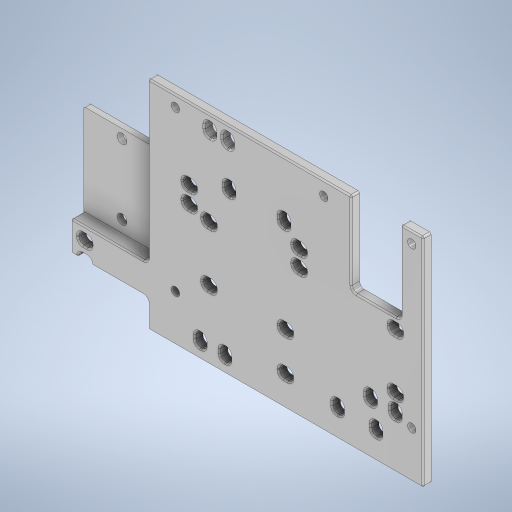
# Autodesk Inventor part: Cable_Fastener_10Gbit
Saved by Autodesk Inventor 2024 (Build 280153000, 153)
## iProperties
Created: 2020-06-16
Part Number: Cable_Fastener_10Gbit
Material: Generic
Document SubType Name: Modeling
Designer: Viktor Lindström
Density: 1 g/cm^3
Appearance: Default
Author: Viktor Lindström
Autodesk Inventor part; units mm, degrees
(part 1 of 2)
ref_plane "YZ Plane" through (0, 0, 0) normal (1, 0, 0) x (0, 1, 0)
ref_plane "XZ Plane" through (0, 0, 0) normal (0, 1, 0) x (-1, 0, 0)
ref_plane "XY Plane" through (0, 0, 0) normal (0, 0, 1) x (1, 0, 0)
sketch "Sketch1" plane through (0, 0, 0) normal (0, 0, 1) x (1, 0, 0)
  line L0 (-50, -39.5) -> (50, -39.5)
  line L1 (50, -39.5) -> (50, 39.5)
  line L2 (50, 39.5) -> (-50, 39.5)
  line L3 (-50, 39.5) -> (-50, -39.5)
  line L4 (-50, -39.5) -> (50, 39.5) construction
  line L5 (50, -39.5) -> (-50, 39.5) construction
  point P0 (0, 0)
  dimension "d0" = 100
  dimension "d1" = 79
  constraints: 12 end point, 2 midpoint, 2 parallel, 1 horizontal, 1 perpendicular
  measures "d0" distance of L1.end L2.end
  measures "d1" distance of L0.end L1.end
extrude "Extrusion1" add sketch "Sketch1" along normal blind 3
sketch "Sketch2" plane through (0, 0, 3) normal (0, 0, 1) x (1, 0, 0)
  circle A0 centre (-40, 35.5) radius 1.5
  circle A1 centre (46, 35.5) radius 1.5
  line L0 (50, 39.5) -> (-50, 39.5) projected
  line L1 (50, -39.5) -> (50, 39.5) projected
  line L2 (-73.7236, 6.5) -> (70.0965, 6.5) construction
  circle A2 centre (-40, -22.5) radius 1.5
  circle A3 centre (46, -22.5) radius 1.5
  point P0 (0, 0)
  dimension "d4" = 3
  dimension "d5" = 3
  dimension "d6" = 86
  dimension "d7" = 4
  dimension "d8" = 4
  dimension "d9" = 4
  dimension "d10" = 33
  constraints: 4 centre point, 2 end point, 2 symmetric about line, 1 horizontal, 2 other
  measures "d4" diameter of A0
  measures "d5" diameter of A1
  measures "d6" distance of A1.centre A0.centre
  measures "d7" distance from line of L0 A1.centre
  measures "d8" distance from line of L0 A0.centre
  measures "d9" distance from line of L1 A1.centre
  measures "d10" distance between parallel lines of L0 L2
extrude "Extrusion2" cut sketch "Sketch2" against normal through all
fillet "Fillet1" radius 0.6 4 edges at (50, 39.5, 1.5) (-50, 39.5, 1.5) (-50, -39.5, 1.5) (50, -39.5, 1.5)
sketch "Sketch3" plane through (0, 0, 3) normal (0, 0, 1) x (1, 0, 0)
  line L0 (31, -32) -> (35, -32)
  line L1 (35, -32) -> (35, -27)
  line L2 (35, -27) -> (31, -27)
  line L3 (31, -27) -> (31, -32)
  line L4 (31, -32) -> (35, -27) construction
  line L5 (35, -32) -> (31, -27) construction
  line L6 (21, -27) -> (17, -27)
  line L7 (17, -27) -> (17, -32)
  line L8 (17, -32) -> (21, -32)
  line L9 (21, -32) -> (21, -27)
  line L10 (21, -27) -> (17, -32) construction
  line L11 (17, -27) -> (21, -32) construction
  line L12 (-2.5, -30.5) -> (2.5, -30.5)
  line L13 (2.5, -30.5) -> (2.5, -26.5)
  line L14 (2.5, -26.5) -> (-2.5, -26.5)
  line L15 (-2.5, -26.5) -> (-2.5, -30.5)
  line L16 (-2.5, -30.5) -> (2.5, -26.5) construction
  line L17 (2.5, -30.5) -> (-2.5, -26.5) construction
  line L18 (-2.5, -12.5) -> (2.5, -12.5)
  line L19 (2.5, -12.5) -> (2.5, -16.5)
  line L20 (2.5, -16.5) -> (-2.5, -16.5)
  line L21 (-2.5, -16.5) -> (-2.5, -12.5)
  line L22 (-2.5, -12.5) -> (2.5, -16.5) construction
  line L23 (2.5, -12.5) -> (-2.5, -16.5) construction
  line L24 (-18.5, 17) -> (-22.5, 17)
  line L25 (-22.5, 17) -> (-22.5, 22)
  line L26 (-22.5, 22) -> (-18.5, 22)
  line L27 (-18.5, 22) -> (-18.5, 17)
  line L28 (-18.5, 17) -> (-22.5, 22) construction
  line L29 (-22.5, 17) -> (-18.5, 22) construction
  line L30 (1.5, 17) -> (-2.5, 17)
  line L31 (-2.5, 17) -> (-2.5, 22)
  line L32 (-2.5, 22) -> (1.5, 22)
  line L33 (1.5, 22) -> (1.5, 17)
  line L34 (1.5, 17) -> (-2.5, 22) construction
  line L35 (-2.5, 17) -> (1.5, 22) construction
  line L36 (37.5, 3.5) -> (42.5, 3.5)
  line L37 (42.5, 3.5) -> (42.5, 7.5)
  line L38 (42.5, 7.5) -> (37.5, 7.5)
  line L39 (37.5, 7.5) -> (37.5, 3.5)
  line L40 (37.5, 3.5) -> (42.5, 7.5) construction
  line L41 (42.5, 3.5) -> (37.5, 7.5) construction
  line L42 (-30.3047, -16.5) -> (-25.3047, -16.5)
  line L43 (-25.3047, -16.5) -> (-25.3047, -12.5)
  line L44 (-25.3047, -12.5) -> (-30.3047, -12.5)
  line L45 (-30.3047, -12.5) -> (-30.3047, -16.5)
  line L46 (-30.3047, -16.5) -> (-25.3047, -12.5) construction
  line L47 (-25.3047, -16.5) -> (-30.3047, -12.5) construction
  line L48 (-25.3047, 3.5) -> (-30.3047, 3.5)
  line L49 (-30.3047, 3.5) -> (-30.3047, 7.5)
  line L50 (-30.3047, 7.5) -> (-25.3047, 7.5)
  line L51 (-25.3047, 7.5) -> (-25.3047, 3.5)
  line L52 (-25.3047, 3.5) -> (-30.3047, 7.5) construction
  line L53 (-30.3047, 3.5) -> (-25.3047, 7.5) construction
  line L54 (50, -38.9) -> (50, 38.9) projected
  line L55 (-49.4, -39.5) -> (49.4, -39.5) projected
  line L56 (49.4, 39.5) -> (-49.4, 39.5) projected
  line L57 (42.5, -16.5) -> (37.5, -16.5)
  line L58 (37.5, -16.5) -> (37.5, -12.5)
  line L59 (37.5, -12.5) -> (42.5, -12.5)
  line L60 (42.5, -12.5) -> (42.5, -16.5)
  line L61 (42.5, -16.5) -> (37.5, -12.5) construction
  line L62 (37.5, -16.5) -> (42.5, -12.5) construction
  line L63 (-50, 38.9) -> (-50, -38.9) projected
  point P0 (0, 0)
  point P1 (33, -29.5)
  point P2 (19, -29.5)
  point P3 (0, -28.5)
  point P4 (0, -14.5)
  point P5 (-20.5, 19.5)
  point P6 (-0.5, 19.5)
  point P7 (40, 5.5)
  point P8 (-27.8047, -14.5)
  point P9 (-27.8047, 5.5)
  point P10 (40, -14.5)
  dimension "d14" = 4
  dimension "d15" = 4
  dimension "d16" = 4
  dimension "d17" = 4
  dimension "d18" = 4
  dimension "d19" = 4
  dimension "d20" = 4
  dimension "d21" = 4
  dimension "d23" = 4
  dimension "d24" = 5
  dimension "d25" = 5
  dimension "d26" = 5
  dimension "d27" = 5
  dimension "d29" = 5
  dimension "d30" = 5
  dimension "d31" = 5
  dimension "d32" = 5
  dimension "d33" = 5
  dimension "d34" = 0
  dimension "d35" = 20
  dimension "d36" = 20
  dimension "d37" = 14
  dimension "d38" = 14
  dimension "d40" = 17
  dimension "d41" = 10
  dimension "d42" = 25
  dimension "d43" = 50
  dimension "d44" = 34
  dimension "d45" = 4
  dimension "d46" = 5
  dimension "d47" = 20
  dimension "d48" = 0
  dimension "d49" = 0
  dimension "d50" = 10
  dimension "d125" = 20
  dimension "d126" = 29.5
  constraints: 120 end point, 20 midpoint, 20 parallel, 10 horizontal, 10 perpendicular, 3 point on line
  measures "d14" distance of L14.end L12.start
  measures "d15" distance of L18.end L19.end
  measures "d16" distance of L44.end L42.start
  measures "d17" distance of L48.end L49.end
  measures "d18" distance of L24.start L24.end
  measures "d19" distance of L30.start L30.end
  measures "d20" distance of L6.start L6.end
  measures "d21" distance of L1.end L2.end
  measures "d23" distance of L38.end L36.start
  measures "d24" distance of L12.start L12.end
  measures "d25" distance of L19.end L20.end
  measures "d26" distance of L6.end L7.end
  measures "d27" distance of L2.end L0.start
  measures "d29" distance of L36.start L36.end
  measures "d30" distance of L32.end L30.start
  measures "d31" distance of L26.end L24.start
  measures "d32" distance of L48.start L48.end
  measures "d33" distance of L42.start L42.end
  measures "d34" vertical distance of point (33, -29.5) point (19, -29.5)
  measures "d35" distance of point (-27.805, 5.5) point (-27.805, -14.5)
  measures "d36" distance of point (-0.5, 19.5) point (-20.5, 19.5)
  measures "d37" distance of point (33, -29.5) point (19, -29.5)
  measures "d38" distance of point (0, -14.5) point (0, -28.5)
  measures "d40" distance from line of L54 point (33, -29.5)
  measures "d41" distance from line of L55 point (33, -29.5)
  measures "d42" distance from line of L55 point (0, -14.5)
  measures "d43" distance from line of L54 point (0, -28.5)
  measures "d44" distance from line of L56 point (-27.805, 5.5)
  measures "d45" distance of L57.end L58.end
  measures "d46" distance of L58.end L59.end
  measures "d47" distance of point (40, 5.5) point (40, -14.5)
  measures "d48" horizontal distance of point (40, 5.5) point (40, -14.5)
  measures "d49" vertical distance of point (40, -14.5) point (-27.805, -14.5)
  measures "d50" distance from line of L54 point (40, -14.5)
  measures "d125" distance from line of L56 point (-20.5, 19.5)
  measures "d126" distance from line of L63 point (-20.5, 19.5)
extrude "Extrusion3" cut sketch "Sketch3" against normal through all
sketch "Sketch4" plane through (0, 0, 3) normal (0, 0, 1) x (1, 0, 0)
  line L0 (-29, -36) -> (-33, -36)
  line L1 (-33, -36) -> (-33, -31)
  line L2 (-33, -31) -> (-29, -31)
  line L3 (-29, -31) -> (-29, -36)
  line L4 (-29, -36) -> (-33, -31) construction
  line L5 (-33, -36) -> (-29, -31) construction
  line L6 (-25.3047, -16.5) -> (-30.3047, -16.5) projected
  line L7 (-30.3047, -12.5) -> (-25.3047, -12.5) projected
  line L8 (-20, -36) -> (-24, -36)
  line L9 (-24, -36) -> (-24, -31)
  line L10 (-24, -31) -> (-20, -31)
  line L11 (-20, -31) -> (-20, -36)
  line L12 (-20, -36) -> (-24, -31) construction
  line L13 (-24, -36) -> (-20, -31) construction
  line L14 (-50, 38.9) -> (-50, -38.9) projected
  line L15 (-49.4, -39.5) -> (49.4, -39.5) projected
  line L16 (32.9777, -23) -> (28.9777, -23)
  line L17 (28.9777, -23) -> (28.9777, -18)
  line L18 (28.9777, -18) -> (32.9777, -18)
  line L19 (32.9777, -18) -> (32.9777, -23)
  line L20 (32.9777, -23) -> (28.9777, -18) construction
  line L21 (28.9777, -23) -> (32.9777, -18) construction
  line L22 (41.9777, -23) -> (37.9777, -23)
  line L23 (37.9777, -23) -> (37.9777, -18)
  line L24 (37.9777, -18) -> (41.9777, -18)
  line L25 (41.9777, -18) -> (41.9777, -23)
  line L26 (41.9777, -23) -> (37.9777, -18) construction
  line L27 (37.9777, -23) -> (41.9777, -18) construction
  line L28 (50, -38.9) -> (50, 38.9) projected
  line L29 (35, -27) -> (35, -32) projected
  line L30 (31, -27) -> (35, -27) projected
  point P0 (0, 0)
  point P1 (-31, -33.5)
  point P2 (-22, -33.5)
  point P3 (30.9777, -20.5)
  point P4 (39.9777, -20.5)
  dimension "d54" = 4
  dimension "d55" = 5
  dimension "d56" = 4
  dimension "d57" = 5
  dimension "d60" = 4
  dimension "d61" = 5
  dimension "d64" = 0
  dimension "d65" = 5
  dimension "d66" = 19
  dimension "d67" = 6
  dimension "d72" = 4
  dimension "d73" = 5
  dimension "d74" = 4
  dimension "d75" = 5
  dimension "d76" = 0
  dimension "d77" = 5
  dimension "d82" = 10.0223
  dimension "d83" = 2.0223
  dimension "d84" = 4
  constraints: 48 end point, 8 midpoint, 8 parallel, 4 horizontal, 4 perpendicular
  measures "d54" distance from line of L7 L6.end
  measures "d55" distance of L6.start L6.end
  measures "d56" distance of L0.start L0.end
  measures "d57" distance of L0.end L1.end
  measures "d60" distance of L8.start L8.end
  measures "d61" distance of L8.end L9.end
  measures "d64" vertical distance of point (-31, -33.5) point (-22, -33.5)
  measures "d65" distance between parallel lines of L3 L9
  measures "d66" distance from line of point (-31, -33.5) L14
  measures "d67" distance from line of L15 point (-31, -33.5)
  measures "d72" distance of L16.start L16.end
  measures "d73" distance of L16.end L17.end
  measures "d74" distance of L25.end L22.end
  measures "d75" distance of L22.end L24.start
  measures "d76" vertical distance of point (30.978, -20.5) point (39.978, -20.5)
  measures "d77" distance between parallel lines of L19 L23
  measures "d82" distance from line of L28 point (39.978, -20.5)
  measures "d83" distance between parallel lines of L29 L19
  measures "d84" distance between parallel lines of L30 L16
extrude "Extrusion4" cut sketch "Sketch4" against normal through all
sketch "Sketch5" plane through (0, 0, 3) normal (0, 0, 1) x (1, 0, 0)
  line L0 (-20, -31) -> (-20, -36) projected
  line L1 (-24, -31) -> (-20, -31) projected
  line L2 (-24, -36) -> (-24, -31) projected
  line L3 (-20, -36) -> (-24, -36) projected
  line L4 (-32.5, 15.5) -> (-37.5, 15.5)
  line L5 (-37.5, 15.5) -> (-37.5, 11.5)
  line L6 (-37.5, 11.5) -> (-32.5, 11.5)
  line L7 (-32.5, 11.5) -> (-32.5, 15.5)
  line L8 (-32.5, 15.5) -> (-37.5, 11.5) construction
  line L9 (-37.5, 15.5) -> (-32.5, 11.5) construction
  line L10 (-37.5, 9.5) -> (-32.5, 9.5)
  line L11 (-32.5, 9.5) -> (-32.5, 5.5)
  line L12 (-32.5, 5.5) -> (-37.5, 5.5)
  line L13 (-37.5, 5.5) -> (-37.5, 9.5)
  line L14 (-37.5, 9.5) -> (-32.5, 5.5) construction
  line L15 (-32.5, 9.5) -> (-37.5, 5.5) construction
  line L16 (49.4, 39.5) -> (-49.4, 39.5) projected
  line L17 (-50, 38.9) -> (-50, -38.9) projected
  line L18 (7.5, 15.5) -> (2.5, 15.5)
  line L19 (2.5, 15.5) -> (2.5, 11.5)
  line L20 (2.5, 11.5) -> (7.5, 11.5)
  line L21 (7.5, 11.5) -> (7.5, 15.5)
  line L22 (7.5, 15.5) -> (2.5, 11.5) construction
  line L23 (2.5, 15.5) -> (7.5, 11.5) construction
  line L24 (2.5, 9.5) -> (7.5, 9.5)
  line L25 (7.5, 9.5) -> (7.5, 5.5)
  line L26 (7.5, 5.5) -> (2.5, 5.5)
  line L27 (2.5, 5.5) -> (2.5, 9.5)
  line L28 (2.5, 9.5) -> (7.5, 5.5) construction
  line L29 (7.5, 9.5) -> (2.5, 5.5) construction
  line L30 (50, -38.9) -> (50, 38.9) projected
  point P0 (-35, 13.5)
  point P1 (-35, 7.5)
  point P2 (5, 13.5)
  point P3 (5, 7.5)
  dimension "d87" = 5
  dimension "d88" = 4
  dimension "d89" = 4
  dimension "d90" = 4
  dimension "d91" = 5
  dimension "d92" = 5
  dimension "d93" = 6
  dimension "d102" = 26
  dimension "d103" = 15
  dimension "d105" = 4
  dimension "d106" = 4
  dimension "d107" = 5
  dimension "d108" = 5
  dimension "d109" = 6
  dimension "d121" = 0
  dimension "d122" = 45
  constraints: 48 end point, 8 midpoint, 8 parallel, 4 horizontal, 4 perpendicular, 2 point on line
  measures "d87" distance of L0.start L0.end
  measures "d88" distance of L1.start L0.start
  measures "d89" distance between parallel lines of L12 L10
  measures "d90" distance of L4.end L5.end
  measures "d91" distance of L10.start L10.end
  measures "d92" distance of L5.end L6.end
  measures "d93" distance of point (-35, 7.5) point (-35, 13.5)
  measures "d102" distance from line of L16 point (-35, 13.5)
  measures "d103" distance from line of L17 point (-35, 13.5)
  measures "d105" distance between parallel lines of L26 L24
  measures "d106" distance of L18.end L19.end
  measures "d107" distance of L24.start L24.end
  measures "d108" distance of L19.end L20.end
  measures "d109" distance of point (5, 7.5) point (5, 13.5)
  measures "d121" distance between parallel lines of L4 L18
  measures "d122" distance from line of L30 point (5, 13.5)
extrude "Extrusion5" cut sketch "Sketch5" against normal through all contours L7 L6 L5 L4 | L10 L11 L12 L13 | L21 L20 L19 L18 | L24 L25 L26 L27
sketch "Sketch6" plane through (0, 0, 3) normal (0, 0, 1) x (1, 0, 0)
  line L0 (49.4, 39.5) -> (-49.4, 39.5) projected
  line L1 (24, 39.5) -> (42, 39.5)
  line L2 (42, 39.5) -> (42, 9.5)
  line L3 (42, 9.5) -> (24, 9.5)
  line L4 (24, 9.5) -> (24, 39.5)
  line L5 (50, -38.9) -> (50, 38.9) projected
  point P0 (0, 0)
  dimension "d127" = 30
  dimension "d128" = 8
  dimension "d129" = 18
  constraints: 8 end point, 2 parallel, 1 horizontal, 1 perpendicular, 1 point on line
  measures "d127" distance between parallel lines of L0 L3
  measures "d128" distance between parallel lines of L5 L2
  measures "d129" distance between parallel lines of L2 L4
extrude "Extrusion6" cut sketch "Sketch6" against normal through all
fillet "Fillet2" radius 0.6 2 edges at (24, 39.5, 1.5) (42, 39.5, 1.5)
fillet "Fillet2" radius 1.75 2 edges at (42, 9.5, 1.5) (24, 9.5, 1.5)
sketch "Sketch7" plane through (0, 0, 3) normal (0, 0, 1) x (1, 0, 0)
  circle A0 centre (-40, -22.5) radius 1.5 projected
  circle A1 centre (-40, 35.5) radius 1.5 projected
  circle A2 centre (46, -22.5) radius 1.5 projected
  circle A3 centre (46, 35.5) radius 1.5 projected
  arc A4 (42.6, 39.5) -> (42, 38.9) centre (42.6, 38.9) ccw projected
  line L0 (42, 38.9) -> (42, 11.25) projected
  line L1 (40.25, 9.5) -> (25.75, 9.5) projected
  line L2 (24, 11.25) -> (24, 38.9) projected
  arc A5 (24, 38.9) -> (23.4, 39.5) centre (23.4, 38.9) ccw projected
  line L3 (23.4, 39.5) -> (-49.4, 39.5) projected
  arc A6 (-49.4, 39.5) -> (-50, 38.9) centre (-49.4, 38.9) ccw projected
  line L4 (-50, 38.9) -> (-50, -38.9) projected
  arc A7 (-50, -38.9) -> (-49.4, -39.5) centre (-49.4, -38.9) ccw projected
  line L5 (-49.4, -39.5) -> (49.4, -39.5) projected
  arc A8 (49.4, -39.5) -> (50, -38.9) centre (49.4, -38.9) ccw projected
  line L6 (50, -38.9) -> (50, 38.9) projected
  arc A9 (50, 38.9) -> (49.4, 39.5) centre (49.4, 38.9) ccw projected
  line L7 (49.4, 39.5) -> (42.6, 39.5) projected
  line L8 (-30.3047, -12.5) -> (-25.3047, -12.5) projected
  line L9 (-25.3047, -12.5) -> (-25.3047, -16.5) projected
  line L10 (-25.3047, -16.5) -> (-30.3047, -16.5) projected
  line L11 (-30.3047, -16.5) -> (-30.3047, -12.5) projected
  line L12 (2.5, -12.5) -> (2.5, -16.5) projected
  line L13 (2.5, -16.5) -> (-2.5, -16.5) projected
  line L14 (-2.5, -16.5) -> (-2.5, -12.5) projected
  line L15 (-2.5, -12.5) -> (2.5, -12.5) projected
  line L16 (37.5, -16.5) -> (37.5, -12.5) projected
  line L17 (37.5, -12.5) -> (42.5, -12.5) projected
  line L18 (42.5, -12.5) -> (42.5, -16.5) projected
  line L19 (42.5, -16.5) -> (37.5, -16.5) projected
  line L20 (31, -27) -> (35, -27) projected
  line L21 (35, -27) -> (35, -32) projected
  line L22 (35, -32) -> (31, -32) projected
  line L23 (31, -32) -> (31, -27) projected
  line L24 (-2.5, 17) -> (-2.5, 22) projected
  line L25 (-2.5, 22) -> (1.5, 22) projected
  line L26 (1.5, 22) -> (1.5, 17) projected
  line L27 (1.5, 17) -> (-2.5, 17) projected
  line L28 (-30.3047, 3.5) -> (-30.3047, 7.5) projected
  line L29 (-30.3047, 7.5) -> (-25.3047, 7.5) projected
  line L30 (-25.3047, 7.5) -> (-25.3047, 3.5) projected
  line L31 (-25.3047, 3.5) -> (-30.3047, 3.5) projected
  line L32 (-2.5, -26.5) -> (2.5, -26.5) projected
  line L33 (2.5, -26.5) -> (2.5, -30.5) projected
  line L34 (2.5, -30.5) -> (-2.5, -30.5) projected
  line L35 (-2.5, -30.5) -> (-2.5, -26.5) projected
  line L36 (37.5, 7.5) -> (42.5, 7.5) projected
  line L37 (42.5, 7.5) -> (42.5, 3.5) projected
  line L38 (42.5, 3.5) -> (37.5, 3.5) projected
  line L39 (37.5, 3.5) -> (37.5, 7.5) projected
  line L40 (21, -32) -> (17, -32) projected
  line L41 (17, -32) -> (17, -27) projected
  line L42 (17, -27) -> (21, -27) projected
  line L43 (21, -27) -> (21, -32) projected
  line L44 (-22.5, 17) -> (-22.5, 22) projected
  line L45 (-22.5, 22) -> (-18.5, 22) projected
  line L46 (-18.5, 22) -> (-18.5, 17) projected
  line L47 (-18.5, 17) -> (-22.5, 17) projected
  line L48 (-24, -36) -> (-24, -31) projected
  line L49 (-24, -31) -> (-20, -31) projected
  line L50 (-20, -31) -> (-20, -36) projected
  line L51 (-20, -36) -> (-24, -36) projected
  line L52 (41.9777, -23) -> (37.9777, -23) projected
  line L53 (37.9777, -23) -> (37.9777, -18) projected
  line L54 (37.9777, -18) -> (41.9777, -18) projected
  line L55 (41.9777, -18) -> (41.9777, -23) projected
  line L56 (-33, -36) -> (-33, -31) projected
  line L57 (-33, -31) -> (-29, -31) projected
  line L58 (-29, -31) -> (-29, -36) projected
  line L59 (-29, -36) -> (-33, -36) projected
  line L60 (28.9777, -23) -> (28.9777, -18) projected
  line L61 (28.9777, -18) -> (32.9777, -18) projected
  line L62 (32.9777, -18) -> (32.9777, -23) projected
  line L63 (32.9777, -23) -> (28.9777, -23) projected
  line L64 (7.5, 11.5) -> (2.5, 11.5) projected
  line L65 (2.5, 11.5) -> (2.5, 15.5) projected
  line L66 (2.5, 15.5) -> (7.5, 15.5) projected
  line L67 (7.5, 15.5) -> (7.5, 11.5) projected
  line L68 (-37.5, 11.5) -> (-37.5, 15.5) projected
  line L69 (-37.5, 15.5) -> (-32.5, 15.5) projected
  line L70 (-32.5, 15.5) -> (-32.5, 11.5) projected
  line L71 (7.5, 9.5) -> (7.5, 5.5) projected
  line L72 (7.5, 5.5) -> (2.5, 5.5) projected
  line L73 (2.5, 5.5) -> (2.5, 9.5) projected
  line L74 (2.5, 9.5) -> (7.5, 9.5) projected
  line L75 (-32.5, 5.5) -> (-37.5, 5.5) projected
  arc A10 (40.25, 9.5) -> (42, 11.25) centre (40.25, 11.25) ccw projected
  arc A11 (24, 11.25) -> (25.75, 9.5) centre (25.75, 11.25) ccw projected
  line L76 (-32.5, 9.5) -> (-32.5, 5.5) projected
  line L77 (-37.5, 5.5) -> (-37.5, 9.5) projected
  line L78 (-37.5, 9.5) -> (-32.5, 9.5) projected
  line L79 (-32.5, 11.5) -> (-37.5, 11.5) projected
  point P0 (0, 0)
fillet "Fillet3" radius 1.75 47 edges at (-37.5, 15.5, 1.5) (-32.5, 15.5, 1.5) (-32.5, 11.5, 1.5) (-37.5, 11.5, 1.5) (-37.5, 5.5, 1.5) (-32.5, 9.5, 1.5) (-37.5, 9.5, 1.5) (-32.5, 5.5, 1.5) (-25.3047, 7.5, 1.5) (-30.3047, 7.5, 1.5) (-30.3047, 3.5, 1.5) (-25.3047, 3.5, 1.5) (-18.5, 17, 1.5) (-22.5, 22, 1.5) (-22.5, 17, 1.5) (-18.5, 22, 1.5) (-2.5, 22, 1.5) (-2.5, 17, 1.5) (1.5, 17, 1.5) (1.5, 22, 1.5) (2.5, 15.5, 1.5) (7.5, 15.5, 1.5) (7.5, 11.5, 1.5) (2.5, 11.5, 1.5) (2.5, 9.5, 1.5) (7.5, 9.5, 1.5) (2.5, 5.5, 1.5) (7.5, 5.5, 1.5) (37.5, 3.5, 1.5) (37.5, 7.5, 1.5) (42.5, 7.5, 1.5) (42.5, 3.5, 1.5) (41.9777, -23, 1.5) (41.9777, -18, 1.5) (42.5, -12.5, 1.5) (37.5, -12.5, 1.5) (28.9777, -18, 1.5) (37.9777, -18, 1.5) (37.9777, -23, 1.5) (28.9777, -23, 1.5) (37.5, -16.5, 1.5) (42.5, -16.5, 1.5) (32.9777, -23, 1.5) (35, -32, 1.5) (35, -27, 1.5) (31, -27, 1.5) (31, -32, 1.5)
fillet "Fillet4" radius 1.75 25 edges at (32.9777, -18, 1.5) (21, -27, 1.5) (21, -32, 1.5) (17, -32, 1.5) (17, -27, 1.5) (-2.5, -12.5, 1.5) (2.5, -12.5, 1.5) (2.5, -16.5, 1.5) (-2.5, -16.5, 1.5) (-2.5, -30.5, 1.5) (-2.5, -26.5, 1.5) (2.5, -26.5, 1.5) (2.5, -30.5, 1.5) (-30.3047, -16.5, 1.5) (-33, -36, 1.5) (-24, -36, 1.5) (-25.3047, -12.5, 1.5) (-29, -31, 1.5) (-20, -31, 1.5) (-30.3047, -12.5, 1.5) (-33, -31, 1.5) (-24, -31, 1.5) (-20, -36, 1.5) (-29, -36, 1.5) (-25.3047, -16.5, 1.5)
sketch "Sketch8" plane through (0, 0, 3) normal (0, 0, 1) x (1, 0, 0)
  circle A0 centre (14, 34.5) radius 1.5
  line L0 (23.4, 39.5) -> (-49.4, 39.5) projected
  line L1 (24, 11.25) -> (24, 38.9) projected
  point P0 (0, 0)
  dimension "d136" = 3
  dimension "d137" = 5
  dimension "d138" = 10
  constraints: 1 centre point
  measures "d136" diameter of A0
  measures "d137" distance from line of L0 A0.centre
  measures "d138" distance from line of L1 A0.centre
extrude "Extrusion7" cut sketch "Sketch8" against normal through all
sketch "Sketch9" plane through (0, 0, 0) normal (0, 0, -1) x (-1, 0, 0)
  circle A0 centre (-14, 34.5) radius 1.5 projected
  arc A1 (-42, 38.9) -> (-42.6, 39.5) centre (-42.6, 38.9) ccw projected
  line L0 (-49.4, 39.5) -> (-42.6, 39.5) projected
  arc A2 (-49.4, 39.5) -> (-50, 38.9) centre (-49.4, 38.9) ccw projected
  line L1 (-50, -38.9) -> (-50, 38.9) projected
  arc A3 (-50, -38.9) -> (-49.4, -39.5) centre (-49.4, -38.9) ccw projected
  line L2 (49.4, -39.5) -> (-49.4, -39.5) projected
  arc A4 (49.4, -39.5) -> (50, -38.9) centre (49.4, -38.9) ccw projected
  line L3 (50, 38.9) -> (50, -38.9) projected
  arc A5 (50, 38.9) -> (49.4, 39.5) centre (49.4, 38.9) ccw projected
  line L4 (-23.4, 39.5) -> (49.4, 39.5) projected
  arc A6 (-23.4, 39.5) -> (-24, 38.9) centre (-23.4, 38.9) ccw projected
  line L5 (-24, 38.9) -> (-24, 11.25) projected
  arc A7 (-25.75, 9.5) -> (-24, 11.25) centre (-25.75, 11.25) ccw projected
  line L6 (-25.75, 9.5) -> (-40.25, 9.5) projected
  arc A8 (-42, 11.25) -> (-40.25, 9.5) centre (-40.25, 11.25) ccw projected
  line L7 (-42, 11.25) -> (-42, 38.9) projected
  line L8 (35.75, 11.5) -> (34.25, 11.5) projected
  arc A9 (32.5, 13.25) -> (34.25, 11.5) centre (34.25, 13.25) ccw projected
  line L9 (32.5, 13.25) -> (32.5, 13.75) projected
  arc A10 (34.25, 15.5) -> (32.5, 13.75) centre (34.25, 13.75) ccw projected
  line L10 (34.25, 15.5) -> (35.75, 15.5) projected
  arc A11 (37.5, 13.75) -> (35.75, 15.5) centre (35.75, 13.75) ccw projected
  line L11 (37.5, 13.75) -> (37.5, 13.25) projected
  arc A12 (35.75, 11.5) -> (37.5, 13.25) centre (35.75, 13.25) ccw projected
  line L12 (-7.5, 7.25) -> (-7.5, 7.75) projected
  arc A13 (-5.75, 9.5) -> (-7.5, 7.75) centre (-5.75, 7.75) ccw projected
  line L13 (-5.75, 9.5) -> (-4.25, 9.5) projected
  arc A14 (-2.5, 7.75) -> (-4.25, 9.5) centre (-4.25, 7.75) ccw projected
  line L14 (-2.5, 7.75) -> (-2.5, 7.25) projected
  arc A15 (-4.25, 5.5) -> (-2.5, 7.25) centre (-4.25, 7.25) ccw projected
  line L15 (-4.25, 5.5) -> (-5.75, 5.5) projected
  arc A16 (-7.5, 7.25) -> (-5.75, 5.5) centre (-5.75, 7.25) ccw projected
  line L16 (32.5, 7.25) -> (32.5, 7.75) projected
  arc A17 (34.25, 9.5) -> (32.5, 7.75) centre (34.25, 7.75) ccw projected
  line L17 (34.25, 9.5) -> (35.75, 9.5) projected
  arc A18 (37.5, 7.75) -> (35.75, 9.5) centre (35.75, 7.75) ccw projected
  line L18 (37.5, 7.75) -> (37.5, 7.25) projected
  arc A19 (35.75, 5.5) -> (37.5, 7.25) centre (35.75, 7.25) ccw projected
  line L19 (35.75, 5.5) -> (34.25, 5.5) projected
  arc A20 (32.5, 7.25) -> (34.25, 5.5) centre (34.25, 7.25) ccw projected
  line L20 (-4.25, 11.5) -> (-5.75, 11.5) projected
  arc A21 (-7.5, 13.25) -> (-5.75, 11.5) centre (-5.75, 13.25) ccw projected
  line L21 (-7.5, 13.25) -> (-7.5, 13.75) projected
  arc A22 (-5.75, 15.5) -> (-7.5, 13.75) centre (-5.75, 13.75) ccw projected
  line L22 (-5.75, 15.5) -> (-4.25, 15.5) projected
  arc A23 (-2.5, 13.75) -> (-4.25, 15.5) centre (-4.25, 13.75) ccw projected
  line L23 (-2.5, 13.75) -> (-2.5, 13.25) projected
  arc A24 (-4.25, 11.5) -> (-2.5, 13.25) centre (-4.25, 13.25) ccw projected
  line L24 (-28.9777, -19.75) -> (-28.9777, -21.25) projected
  arc A25 (-30.7277, -23) -> (-28.9777, -21.25) centre (-30.7277, -21.25) ccw projected
  line L25 (-30.7277, -23) -> (-31.2277, -23) projected
  arc A26 (-32.9777, -21.25) -> (-31.2277, -23) centre (-31.2277, -21.25) ccw projected
  line L26 (-32.9777, -21.25) -> (-32.9777, -19.75) projected
  arc A27 (-31.2277, -18) -> (-32.9777, -19.75) centre (-31.2277, -19.75) ccw projected
  line L27 (-31.2277, -18) -> (-30.7277, -18) projected
  arc A28 (-28.9777, -19.75) -> (-30.7277, -18) centre (-30.7277, -19.75) ccw projected
  line L28 (33, -32.75) -> (33, -34.25) projected
  arc A29 (31.25, -36) -> (33, -34.25) centre (31.25, -34.25) ccw projected
  line L29 (31.25, -36) -> (30.75, -36) projected
  arc A30 (29, -34.25) -> (30.75, -36) centre (30.75, -34.25) ccw projected
  line L30 (29, -34.25) -> (29, -32.75) projected
  arc A31 (30.75, -31) -> (29, -32.75) centre (30.75, -32.75) ccw projected
  line L31 (30.75, -31) -> (31.25, -31) projected
  arc A32 (33, -32.75) -> (31.25, -31) centre (31.25, -32.75) ccw projected
  line L32 (-39.7277, -23) -> (-40.2277, -23) projected
  arc A33 (-41.9777, -21.25) -> (-40.2277, -23) centre (-40.2277, -21.25) ccw projected
  line L33 (-41.9777, -21.25) -> (-41.9777, -19.75) projected
  arc A34 (-40.2277, -18) -> (-41.9777, -19.75) centre (-40.2277, -19.75) ccw projected
  line L34 (-40.2277, -18) -> (-39.7277, -18) projected
  arc A35 (-37.9777, -19.75) -> (-39.7277, -18) centre (-39.7277, -19.75) ccw projected
  line L35 (-37.9777, -19.75) -> (-37.9777, -21.25) projected
  arc A36 (-39.7277, -23) -> (-37.9777, -21.25) centre (-39.7277, -21.25) ccw projected
  line L36 (24, -32.75) -> (24, -34.25) projected
  arc A37 (22.25, -36) -> (24, -34.25) centre (22.25, -34.25) ccw projected
  line L37 (22.25, -36) -> (21.75, -36) projected
  arc A38 (20, -34.25) -> (21.75, -36) centre (21.75, -34.25) ccw projected
  line L38 (20, -34.25) -> (20, -32.75) projected
  arc A39 (21.75, -31) -> (20, -32.75) centre (21.75, -32.75) ccw projected
  line L39 (21.75, -31) -> (22.25, -31) projected
  arc A40 (24, -32.75) -> (22.25, -31) centre (22.25, -32.75) ccw projected
  line L40 (22.5, 20.25) -> (22.5, 18.75) projected
  arc A41 (20.75, 17) -> (22.5, 18.75) centre (20.75, 18.75) ccw projected
  line L41 (20.75, 17) -> (20.25, 17) projected
  arc A42 (18.5, 18.75) -> (20.25, 17) centre (20.25, 18.75) ccw projected
  line L42 (18.5, 18.75) -> (18.5, 20.25) projected
  arc A43 (20.25, 22) -> (18.5, 20.25) centre (20.25, 20.25) ccw projected
  line L43 (20.25, 22) -> (20.75, 22) projected
  arc A44 (22.5, 20.25) -> (20.75, 22) centre (20.75, 20.25) ccw projected
  line L44 (-18.75, -32) -> (-19.25, -32) projected
  arc A45 (-21, -30.25) -> (-19.25, -32) centre (-19.25, -30.25) ccw projected
  line L45 (-21, -30.25) -> (-21, -28.75) projected
  arc A46 (-19.25, -27) -> (-21, -28.75) centre (-19.25, -28.75) ccw projected
  line L46 (-19.25, -27) -> (-18.75, -27) projected
  arc A47 (-17, -28.75) -> (-18.75, -27) centre (-18.75, -28.75) ccw projected
  line L47 (-17, -28.75) -> (-17, -30.25) projected
  arc A48 (-18.75, -32) -> (-17, -30.25) centre (-18.75, -30.25) ccw projected
  line L48 (-40.75, 7.5) -> (-39.25, 7.5) projected
  arc A49 (-37.5, 5.75) -> (-39.25, 7.5) centre (-39.25, 5.75) ccw projected
  line L49 (-37.5, 5.75) -> (-37.5, 5.25) projected
  arc A50 (-39.25, 3.5) -> (-37.5, 5.25) centre (-39.25, 5.25) ccw projected
  line L50 (-39.25, 3.5) -> (-40.75, 3.5) projected
  arc A51 (-42.5, 5.25) -> (-40.75, 3.5) centre (-40.75, 5.25) ccw projected
  line L51 (-42.5, 5.25) -> (-42.5, 5.75) projected
  arc A52 (-40.75, 7.5) -> (-42.5, 5.75) centre (-40.75, 5.75) ccw projected
  line L52 (-0.75, -26.5) -> (0.75, -26.5) projected
  arc A53 (2.5, -28.25) -> (0.75, -26.5) centre (0.75, -28.25) ccw projected
  line L53 (2.5, -28.25) -> (2.5, -28.75) projected
  arc A54 (0.75, -30.5) -> (2.5, -28.75) centre (0.75, -28.75) ccw projected
  line L54 (0.75, -30.5) -> (-0.75, -30.5) projected
  arc A55 (-2.5, -28.75) -> (-0.75, -30.5) centre (-0.75, -28.75) ccw projected
  line L55 (-2.5, -28.75) -> (-2.5, -28.25) projected
  arc A56 (-0.75, -26.5) -> (-2.5, -28.25) centre (-0.75, -28.25) ccw projected
  line L56 (30.3047, 5.75) -> (30.3047, 5.25) projected
  arc A57 (28.5547, 3.5) -> (30.3047, 5.25) centre (28.5547, 5.25) ccw projected
  line L57 (28.5547, 3.5) -> (27.0547, 3.5) projected
  arc A58 (25.3047, 5.25) -> (27.0547, 3.5) centre (27.0547, 5.25) ccw projected
  line L58 (25.3047, 5.25) -> (25.3047, 5.75) projected
  arc A59 (27.0547, 7.5) -> (25.3047, 5.75) centre (27.0547, 5.75) ccw projected
  line L59 (27.0547, 7.5) -> (28.5547, 7.5) projected
  arc A60 (30.3047, 5.75) -> (28.5547, 7.5) centre (28.5547, 5.75) ccw projected
  line L60 (2.5, 20.25) -> (2.5, 18.75) projected
  arc A61 (0.75, 17) -> (2.5, 18.75) centre (0.75, 18.75) ccw projected
  line L61 (0.75, 17) -> (0.25, 17) projected
  arc A62 (-1.5, 18.75) -> (0.25, 17) centre (0.25, 18.75) ccw projected
  line L62 (-1.5, 18.75) -> (-1.5, 20.25) projected
  arc A63 (0.25, 22) -> (-1.5, 20.25) centre (0.25, 20.25) ccw projected
  line L63 (0.25, 22) -> (0.75, 22) projected
  arc A64 (2.5, 20.25) -> (0.75, 22) centre (0.75, 20.25) ccw projected
  line L64 (-33.25, -27) -> (-32.75, -27) projected
  arc A65 (-31, -28.75) -> (-32.75, -27) centre (-32.75, -28.75) ccw projected
  line L65 (-31, -28.75) -> (-31, -30.25) projected
  arc A66 (-32.75, -32) -> (-31, -30.25) centre (-32.75, -30.25) ccw projected
  line L66 (-32.75, -32) -> (-33.25, -32) projected
  arc A67 (-35, -30.25) -> (-33.25, -32) centre (-33.25, -30.25) ccw projected
  line L67 (-35, -30.25) -> (-35, -28.75) projected
  arc A68 (-33.25, -27) -> (-35, -28.75) centre (-33.25, -28.75) ccw projected
  line L68 (-37.5, -14.25) -> (-37.5, -14.75) projected
  arc A69 (-39.25, -16.5) -> (-37.5, -14.75) centre (-39.25, -14.75) ccw projected
  line L69 (-39.25, -16.5) -> (-40.75, -16.5) projected
  arc A70 (-42.5, -14.75) -> (-40.75, -16.5) centre (-40.75, -14.75) ccw projected
  line L70 (-42.5, -14.75) -> (-42.5, -14.25) projected
  arc A71 (-40.75, -12.5) -> (-42.5, -14.25) centre (-40.75, -14.25) ccw projected
  line L71 (-40.75, -12.5) -> (-39.25, -12.5) projected
  arc A72 (-37.5, -14.25) -> (-39.25, -12.5) centre (-39.25, -14.25) ccw projected
  line L72 (-2.5, -14.75) -> (-2.5, -14.25) projected
  arc A73 (-0.75, -12.5) -> (-2.5, -14.25) centre (-0.75, -14.25) ccw projected
  line L73 (-0.75, -12.5) -> (0.75, -12.5) projected
  arc A74 (2.5, -14.25) -> (0.75, -12.5) centre (0.75, -14.25) ccw projected
  line L74 (2.5, -14.25) -> (2.5, -14.75) projected
  arc A75 (0.75, -16.5) -> (2.5, -14.75) centre (0.75, -14.75) ccw projected
  line L75 (0.75, -16.5) -> (-0.75, -16.5) projected
  arc A76 (-2.5, -14.75) -> (-0.75, -16.5) centre (-0.75, -14.75) ccw projected
  line L76 (27.0547, -12.5) -> (28.5547, -12.5) projected
  arc A77 (30.3047, -14.25) -> (28.5547, -12.5) centre (28.5547, -14.25) ccw projected
  line L77 (30.3047, -14.25) -> (30.3047, -14.75) projected
  arc A78 (28.5547, -16.5) -> (30.3047, -14.75) centre (28.5547, -14.75) ccw projected
  line L78 (28.5547, -16.5) -> (27.0547, -16.5) projected
  arc A79 (25.3047, -14.75) -> (27.0547, -16.5) centre (27.0547, -14.75) ccw projected
  line L79 (25.3047, -14.75) -> (25.3047, -14.25) projected
  arc A80 (27.0547, -12.5) -> (25.3047, -14.25) centre (27.0547, -14.25) ccw projected
  circle A81 centre (-46, 35.5) radius 1.5 projected
  circle A82 centre (-46, -22.5) radius 1.5 projected
  circle A83 centre (40, 35.5) radius 1.5 projected
  circle A84 centre (40, -22.5) radius 1.5 projected
  line L80 (37.8, -11) -> (-3.2, -11)
  line L81 (-3.2, -11) -> (-3.2, -3)
  line L82 (-3.2, -3) -> (37.8, -3)
  line L83 (37.8, -3) -> (37.8, -11)
  point P0 (0, 0)
  point P1 (-3.2, -7)
  point P2 (25.8299, 4)
  point P3 (29.7794, 4)
  point P4 (37.8, -7)
  dimension "d145" = 8
  dimension "d146" = 12.2
  dimension "d147" = 41
  dimension "d151" = 28.5
  constraints: 8 end point, 2 midpoint, 2 parallel, 1 horizontal, 1 perpendicular
  measures "d145" distance between parallel lines of L82 L80
  measures "d146" distance between parallel lines of L3 L83
  measures "d147" distance from line of point (-3.2, -7) L83
  measures "d151" distance between parallel lines of L2 L80
extrude "Extrusion8" cut sketch "Sketch9" against normal blind 1.5 contours L80 L81 L82 L83
fillet "Fillet5" radius 1.75 4 edges at (-37.8, -3, 0.75) (-37.8, -11, 0.75) (3.2, -11, 0.75) (3.2, -3, 0.75)
sketch "Sketch10" plane through (0, 0, 0) normal (0, 0, -1) x (-1, 0, 0)
  line L0 (-3.2, -9.25) -> (-3.2, -4.75) projected
  line L1 (-3.2, -7) -> (-17.1515, -7) construction
  line L2 (-36.2, 3.5) -> (-3.2, 3.5)
  line L3 (-3.2, 3.5) -> (-3.2, -17.5)
  line L4 (-3.2, -17.5) -> (-36.2, -17.5)
  line L5 (-36.2, -17.5) -> (-36.2, 3.5)
  line L6 (-36.2, 3.5) -> (-3.2, -17.5) construction
  line L7 (-3.2, 3.5) -> (-36.2, -17.5) construction
  line L8 (-3.2, -9.25) -> (-3.2, -4.75) projected
  point P0 (0, 0)
  point P1 (-19.7, -7)
  point P2 (-3.2, -7)
  dimension "d153" = 21
  dimension "d154" = 33
  constraints: 14 end point, 5 midpoint, 2 horizontal, 2 parallel, 1 perpendicular, 1 point on line
  measures "d153" distance between parallel lines of L4 L2
  measures "d154" distance between parallel lines of L3 L5
extrude "Extrusion9" add sketch "Sketch10" along normal blind 2.25
fillet "Fillet6" radius 1.75 4 edges at (3.2, -17.5, -1.125) (36.2, -17.5, -1.125) (36.2, 3.5, -1.125) (3.2, 3.5, -1.125)
sketch "Sketch11" plane through (0, 0, 0) normal (0, 0, -1) x (-1, 0, 0)
  circle A0 centre (40, -22.5) radius 1.5 projected
  circle A1 centre (40, 35.5) radius 1.5 projected
  circle A2 centre (-46, -22.5) radius 1.5 projected
  circle A3 centre (-46, 35.5) radius 1.5 projected
  line L0 (27.0547, -12.5) -> (28.5547, -12.5) projected
  arc A4 (30.3047, -14.25) -> (28.5547, -12.5) centre (28.5547, -14.25) ccw projected
  line L1 (30.3047, -14.25) -> (30.3047, -14.75) projected
  arc A5 (28.5547, -16.5) -> (30.3047, -14.75) centre (28.5547, -14.75) ccw projected
  line L2 (28.5547, -16.5) -> (27.0547, -16.5) projected
  arc A6 (25.3047, -14.75) -> (27.0547, -16.5) centre (27.0547, -14.75) ccw projected
  line L3 (25.3047, -14.75) -> (25.3047, -14.25) projected
  arc A7 (27.0547, -12.5) -> (25.3047, -14.25) centre (27.0547, -14.25) ccw projected
  line L4 (-2.5, -14.75) -> (-2.5, -14.25) projected
  arc A8 (-0.75, -12.5) -> (-2.5, -14.25) centre (-0.75, -14.25) ccw projected
  line L5 (-0.75, -12.5) -> (0.75, -12.5) projected
  arc A9 (2.5, -14.25) -> (0.75, -12.5) centre (0.75, -14.25) ccw projected
  line L6 (2.5, -14.25) -> (2.5, -14.75) projected
  arc A10 (0.75, -16.5) -> (2.5, -14.75) centre (0.75, -14.75) ccw projected
  line L7 (0.75, -16.5) -> (-0.75, -16.5) projected
  arc A11 (-2.5, -14.75) -> (-0.75, -16.5) centre (-0.75, -14.75) ccw projected
  line L8 (-37.5, -14.25) -> (-37.5, -14.75) projected
  arc A12 (-39.25, -16.5) -> (-37.5, -14.75) centre (-39.25, -14.75) ccw projected
  line L9 (-39.25, -16.5) -> (-40.75, -16.5) projected
  arc A13 (-42.5, -14.75) -> (-40.75, -16.5) centre (-40.75, -14.75) ccw projected
  line L10 (-42.5, -14.75) -> (-42.5, -14.25) projected
  arc A14 (-40.75, -12.5) -> (-42.5, -14.25) centre (-40.75, -14.25) ccw projected
  line L11 (-40.75, -12.5) -> (-39.25, -12.5) projected
  arc A15 (-37.5, -14.25) -> (-39.25, -12.5) centre (-39.25, -14.25) ccw projected
  line L12 (-33.25, -27) -> (-32.75, -27) projected
  arc A16 (-31, -28.75) -> (-32.75, -27) centre (-32.75, -28.75) ccw projected
  line L13 (-31, -28.75) -> (-31, -30.25) projected
  arc A17 (-32.75, -32) -> (-31, -30.25) centre (-32.75, -30.25) ccw projected
  line L14 (-32.75, -32) -> (-33.25, -32) projected
  arc A18 (-35, -30.25) -> (-33.25, -32) centre (-33.25, -30.25) ccw projected
  line L15 (-35, -30.25) -> (-35, -28.75) projected
  arc A19 (-33.25, -27) -> (-35, -28.75) centre (-33.25, -28.75) ccw projected
  line L16 (2.5, 20.25) -> (2.5, 18.75) projected
  arc A20 (0.75, 17) -> (2.5, 18.75) centre (0.75, 18.75) ccw projected
  line L17 (0.75, 17) -> (0.25, 17) projected
  arc A21 (-1.5, 18.75) -> (0.25, 17) centre (0.25, 18.75) ccw projected
  line L18 (-1.5, 18.75) -> (-1.5, 20.25) projected
  arc A22 (0.25, 22) -> (-1.5, 20.25) centre (0.25, 20.25) ccw projected
  line L19 (0.25, 22) -> (0.75, 22) projected
  arc A23 (2.5, 20.25) -> (0.75, 22) centre (0.75, 20.25) ccw projected
  line L20 (30.3047, 5.75) -> (30.3047, 5.25) projected
  arc A24 (28.5547, 3.5) -> (30.3047, 5.25) centre (28.5547, 5.25) ccw projected
  line L21 (28.5547, 3.5) -> (27.0547, 3.5) projected
  arc A25 (25.3047, 5.25) -> (27.0547, 3.5) centre (27.0547, 5.25) ccw projected
  line L22 (25.3047, 5.25) -> (25.3047, 5.75) projected
  arc A26 (27.0547, 7.5) -> (25.3047, 5.75) centre (27.0547, 5.75) ccw projected
  line L23 (27.0547, 7.5) -> (28.5547, 7.5) projected
  arc A27 (30.3047, 5.75) -> (28.5547, 7.5) centre (28.5547, 5.75) ccw projected
  line L24 (-0.75, -26.5) -> (0.75, -26.5) projected
  arc A28 (2.5, -28.25) -> (0.75, -26.5) centre (0.75, -28.25) ccw projected
  line L25 (2.5, -28.25) -> (2.5, -28.75) projected
  arc A29 (0.75, -30.5) -> (2.5, -28.75) centre (0.75, -28.75) ccw projected
  line L26 (0.75, -30.5) -> (-0.75, -30.5) projected
  arc A30 (-2.5, -28.75) -> (-0.75, -30.5) centre (-0.75, -28.75) ccw projected
  line L27 (-2.5, -28.75) -> (-2.5, -28.25) projected
  arc A31 (-0.75, -26.5) -> (-2.5, -28.25) centre (-0.75, -28.25) ccw projected
  line L28 (-40.75, 7.5) -> (-39.25, 7.5) projected
  arc A32 (-37.5, 5.75) -> (-39.25, 7.5) centre (-39.25, 5.75) ccw projected
  line L29 (-37.5, 5.75) -> (-37.5, 5.25) projected
  arc A33 (-39.25, 3.5) -> (-37.5, 5.25) centre (-39.25, 5.25) ccw projected
  line L30 (-39.25, 3.5) -> (-40.75, 3.5) projected
  arc A34 (-42.5, 5.25) -> (-40.75, 3.5) centre (-40.75, 5.25) ccw projected
  line L31 (-42.5, 5.25) -> (-42.5, 5.75) projected
  arc A35 (-40.75, 7.5) -> (-42.5, 5.75) centre (-40.75, 5.75) ccw projected
  line L32 (-18.75, -32) -> (-19.25, -32) projected
  arc A36 (-21, -30.25) -> (-19.25, -32) centre (-19.25, -30.25) ccw projected
  line L33 (-21, -30.25) -> (-21, -28.75) projected
  arc A37 (-19.25, -27) -> (-21, -28.75) centre (-19.25, -28.75) ccw projected
  line L34 (-19.25, -27) -> (-18.75, -27) projected
  arc A38 (-17, -28.75) -> (-18.75, -27) centre (-18.75, -28.75) ccw projected
  line L35 (-17, -28.75) -> (-17, -30.25) projected
  arc A39 (-18.75, -32) -> (-17, -30.25) centre (-18.75, -30.25) ccw projected
  line L36 (22.5, 20.25) -> (22.5, 18.75) projected
  arc A40 (20.75, 17) -> (22.5, 18.75) centre (20.75, 18.75) ccw projected
  line L37 (20.75, 17) -> (20.25, 17) projected
  arc A41 (18.5, 18.75) -> (20.25, 17) centre (20.25, 18.75) ccw projected
  line L38 (18.5, 18.75) -> (18.5, 20.25) projected
  arc A42 (20.25, 22) -> (18.5, 20.25) centre (20.25, 20.25) ccw projected
  line L39 (20.25, 22) -> (20.75, 22) projected
  arc A43 (22.5, 20.25) -> (20.75, 22) centre (20.75, 20.25) ccw projected
  line L40 (24, -32.75) -> (24, -34.25) projected
  arc A44 (22.25, -36) -> (24, -34.25) centre (22.25, -34.25) ccw projected
  line L41 (22.25, -36) -> (21.75, -36) projected
  arc A45 (20, -34.25) -> (21.75, -36) centre (21.75, -34.25) ccw projected
  line L42 (20, -34.25) -> (20, -32.75) projected
  arc A46 (21.75, -31) -> (20, -32.75) centre (21.75, -32.75) ccw projected
  line L43 (21.75, -31) -> (22.25, -31) projected
  arc A47 (24, -32.75) -> (22.25, -31) centre (22.25, -32.75) ccw projected
  line L44 (-39.7277, -23) -> (-40.2277, -23) projected
  arc A48 (-41.9777, -21.25) -> (-40.2277, -23) centre (-40.2277, -21.25) ccw projected
  line L45 (-41.9777, -21.25) -> (-41.9777, -19.75) projected
  arc A49 (-40.2277, -18) -> (-41.9777, -19.75) centre (-40.2277, -19.75) ccw projected
  line L46 (-40.2277, -18) -> (-39.7277, -18) projected
  arc A50 (-37.9777, -19.75) -> (-39.7277, -18) centre (-39.7277, -19.75) ccw projected
  line L47 (-37.9777, -19.75) -> (-37.9777, -21.25) projected
  arc A51 (-39.7277, -23) -> (-37.9777, -21.25) centre (-39.7277, -21.25) ccw projected
  line L48 (33, -32.75) -> (33, -34.25) projected
  arc A52 (31.25, -36) -> (33, -34.25) centre (31.25, -34.25) ccw projected
  line L49 (31.25, -36) -> (30.75, -36) projected
  arc A53 (29, -34.25) -> (30.75, -36) centre (30.75, -34.25) ccw projected
  line L50 (29, -34.25) -> (29, -32.75) projected
  arc A54 (30.75, -31) -> (29, -32.75) centre (30.75, -32.75) ccw projected
  line L51 (30.75, -31) -> (31.25, -31) projected
  arc A55 (33, -32.75) -> (31.25, -31) centre (31.25, -32.75) ccw projected
  line L52 (-28.9777, -19.75) -> (-28.9777, -21.25) projected
  arc A56 (-30.7277, -23) -> (-28.9777, -21.25) centre (-30.7277, -21.25) ccw projected
  line L53 (-30.7277, -23) -> (-31.2277, -23) projected
  arc A57 (-32.9777, -21.25) -> (-31.2277, -23) centre (-31.2277, -21.25) ccw projected
  line L54 (-32.9777, -21.25) -> (-32.9777, -19.75) projected
  arc A58 (-31.2277, -18) -> (-32.9777, -19.75) centre (-31.2277, -19.75) ccw projected
  line L55 (-31.2277, -18) -> (-30.7277, -18) projected
  arc A59 (-28.9777, -19.75) -> (-30.7277, -18) centre (-30.7277, -19.75) ccw projected
  line L56 (-4.25, 11.5) -> (-5.75, 11.5) projected
  arc A60 (-7.5, 13.25) -> (-5.75, 11.5) centre (-5.75, 13.25) ccw projected
  line L57 (-7.5, 13.25) -> (-7.5, 13.75) projected
  arc A61 (-5.75, 15.5) -> (-7.5, 13.75) centre (-5.75, 13.75) ccw projected
  line L58 (-5.75, 15.5) -> (-4.25, 15.5) projected
  arc A62 (-2.5, 13.75) -> (-4.25, 15.5) centre (-4.25, 13.75) ccw projected
  line L59 (-2.5, 13.75) -> (-2.5, 13.25) projected
  arc A63 (-4.25, 11.5) -> (-2.5, 13.25) centre (-4.25, 13.25) ccw projected
  line L60 (32.5, 7.25) -> (32.5, 7.75) projected
  arc A64 (34.25, 9.5) -> (32.5, 7.75) centre (34.25, 7.75) ccw projected
  line L61 (34.25, 9.5) -> (35.75, 9.5) projected
  arc A65 (37.5, 7.75) -> (35.75, 9.5) centre (35.75, 7.75) ccw projected
  line L62 (37.5, 7.75) -> (37.5, 7.25) projected
  arc A66 (35.75, 5.5) -> (37.5, 7.25) centre (35.75, 7.25) ccw projected
  line L63 (35.75, 5.5) -> (34.25, 5.5) projected
  arc A67 (32.5, 7.25) -> (34.25, 5.5) centre (34.25, 7.25) ccw projected
  line L64 (-7.5, 7.25) -> (-7.5, 7.75) projected
  arc A68 (-5.75, 9.5) -> (-7.5, 7.75) centre (-5.75, 7.75) ccw projected
  line L65 (-5.75, 9.5) -> (-4.25, 9.5) projected
  arc A69 (-2.5, 7.75) -> (-4.25, 9.5) centre (-4.25, 7.75) ccw projected
  line L66 (-2.5, 7.75) -> (-2.5, 7.25) projected
  arc A70 (-4.25, 5.5) -> (-2.5, 7.25) centre (-4.25, 7.25) ccw projected
  line L67 (-4.25, 5.5) -> (-5.75, 5.5) projected
  arc A71 (-7.5, 7.25) -> (-5.75, 5.5) centre (-5.75, 7.25) ccw projected
  line L68 (35.75, 11.5) -> (34.25, 11.5) projected
  arc A72 (32.5, 13.25) -> (34.25, 11.5) centre (34.25, 13.25) ccw projected
  line L69 (32.5, 13.25) -> (32.5, 13.75) projected
  arc A73 (34.25, 15.5) -> (32.5, 13.75) centre (34.25, 13.75) ccw projected
  line L70 (34.25, 15.5) -> (35.75, 15.5) projected
  arc A74 (37.5, 13.75) -> (35.75, 15.5) centre (35.75, 13.75) ccw projected
  line L71 (37.5, 13.75) -> (37.5, 13.25) projected
  arc A75 (35.75, 11.5) -> (37.5, 13.25) centre (35.75, 13.25) ccw projected
  arc A76 (-42, 38.9) -> (-42.6, 39.5) centre (-42.6, 38.9) ccw projected
  line L72 (-49.4, 39.5) -> (-42.6, 39.5) projected
  arc A77 (-49.4, 39.5) -> (-50, 38.9) centre (-49.4, 38.9) ccw projected
  line L73 (-50, -38.9) -> (-50, 38.9) projected
  arc A78 (-50, -38.9) -> (-49.4, -39.5) centre (-49.4, -38.9) ccw projected
  line L74 (49.4, -39.5) -> (-49.4, -39.5) projected
  arc A79 (49.4, -39.5) -> (50, -38.9) centre (49.4, -38.9) ccw projected
  line L75 (50, 38.9) -> (50, -38.9) projected
  arc A80 (50, 38.9) -> (49.4, 39.5) centre (49.4, 38.9) ccw projected
  line L76 (-23.4, 39.5) -> (49.4, 39.5) projected
  arc A81 (-23.4, 39.5) -> (-24, 38.9) centre (-23.4, 38.9) ccw projected
  line L77 (-24, 38.9) -> (-24, 11.25) projected
  arc A82 (-25.75, 9.5) -> (-24, 11.25) centre (-25.75, 11.25) ccw projected
  line L78 (-25.75, 9.5) -> (-40.25, 9.5) projected
  arc A83 (-42, 11.25) -> (-40.25, 9.5) centre (-40.25, 11.25) ccw projected
  line L79 (-42, 11.25) -> (-42, 38.9) projected
  circle A84 centre (-14, 34.5) radius 1.5 projected
  line L80 (-3.2, -9.25) -> (-3.2, -15.75) projected
  arc A85 (-4.95, -17.5) -> (-3.2, -15.75) centre (-4.95, -15.75) ccw projected
  line L81 (-4.95, -17.5) -> (-34.45, -17.5) projected
  arc A86 (-36.2, -15.75) -> (-34.45, -17.5) centre (-34.45, -15.75) ccw projected
  line L82 (-36.2, -15.75) -> (-36.2, 1.75) projected
  arc A87 (-34.45, 3.5) -> (-36.2, 1.75) centre (-34.45, 1.75) ccw projected
  line L83 (-34.45, 3.5) -> (-4.95, 3.5) projected
  arc A88 (-3.2, 1.75) -> (-4.95, 3.5) centre (-4.95, 1.75) ccw projected
  line L84 (-3.2, 1.75) -> (-3.2, -4.75) projected
  arc A89 (-1.45, -3) -> (-3.2, -4.75) centre (-1.45, -4.75) ccw projected
  line L85 (-1.45, -3) -> (36.05, -3) projected
  arc A90 (37.8, -4.75) -> (36.05, -3) centre (36.05, -4.75) ccw projected
  line L86 (37.8, -4.75) -> (37.8, -9.25) projected
  arc A91 (36.05, -11) -> (37.8, -9.25) centre (36.05, -9.25) ccw projected
  line L87 (36.05, -11) -> (-1.45, -11) projected
  arc A92 (-3.2, -9.25) -> (-1.45, -11) centre (-1.45, -9.25) ccw projected
  line L88 (47, -39.5) -> (78, -39.5)
  line L89 (78, -39.5) -> (78, 14.5)
  line L90 (78, 14.5) -> (47, 14.5)
  line L91 (47, 14.5) -> (47, -39.5)
  line L92 (50, 38.9) -> (50, -38.9) projected
  point P0 (0, 0)
  point P1 (50, 14.5)
  dimension "d158" = 54
  dimension "d159" = 3
  dimension "d160" = 28
  constraints: 8 end point, 2 parallel, 1 horizontal, 1 perpendicular, 1 point on line
  measures "d158" distance of L88.end L89.end
  measures "d159" distance between parallel lines of L75 L91
  measures "d160" distance between parallel lines of L92 L89
extrude "Extrusion10" add sketch "Sketch11" against normal up to surface (3 mm away) contours A79 L75 L90 L89 L88
extrude "Extrusion11" add sketch "Sketch11" along normal blind 3.6 contours L91 L90 L75 A79 L74 | A79 L75 L90 L89 L88